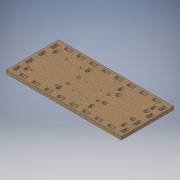
# Autodesk Inventor part: case_base
Saved by Autodesk Inventor 2019 (Build 230136000, 136)
## iProperties
Created: 2019-02-02
Part Number: case_base
Material: MDF Medium Density Fiberboard
Document SubType Name: Modeling
Designer: suchanek
Density: 0.8 g/cm^3
Appearance: Cardboard - Corrugated
Author: suchanek
Autodesk Inventor part; units mm, degrees
ref_plane "YZ Plane" through (0, 0, 0) normal (1, 0, 0) x (0, 1, 0)
ref_plane "XZ Plane" through (0, 0, 0) normal (0, 1, 0) x (-1, 0, 0)
ref_plane "XY Plane" through (0, 0, 0) normal (0, 0, 1) x (1, 0, 0)
sketch "Sketch1" plane through (0, 0, 0) normal (0, 1, 0) x (-1, 0, 0)
  line L0 (110, 50) -> (-110, 50)
  line L1 (-110, 50) -> (-110, -50)
  line L2 (-110, -50) -> (110, -50)
  line L3 (110, -50) -> (110, 50)
  line L4 (110, 50) -> (-110, -50) construction
  line L5 (-110, 50) -> (110, -50) construction
  circle A0 centre (-13.5, 20) radius 0.9
  circle A1 centre (13.5, 20) radius 0.9
  circle A2 centre (13.5, -7) radius 0.9
  circle A3 centre (-13.5, -7) radius 0.9
  line L6 (-13.5, 20) -> (13.5, 20)
  line L7 (13.5, -7) -> (-13.5, -7)
  line L8 (0, 0) -> (4.5236, 0)
  circle A4 centre (28.5, -7) radius 2.6
  circle A5 centre (-28.5, -7) radius 2.6
  circle A6 centre (28.5, 13.5) radius 2.6
  circle A7 centre (-28.5, 13.5) radius 2.6
  line L9 (0, -7) -> (0, -18)
  circle A8 centre (70.5, -25.1) radius 1.6
  circle A9 centre (42.6, -25.1) radius 1.6
  circle A10 centre (85.7, 25.7) radius 1.6
  circle A11 centre (37.5, 27) radius 1.6
  circle A12 centre (-38.5, -16) radius 4
  circle A13 centre (-38.5, 10) radius 4
  circle A14 centre (-92, 10) radius 4
  circle A15 centre (-92, -16) radius 4
  circle A16 centre (31, 28) radius 2.6
  circle A17 centre (31, -28) radius 2.6
  line L10 (0, 0) -> (5.2635, 0)
  circle A18 centre (-31, 28) radius 2.6
  circle A19 centre (-31, -28) radius 2.6
  line L11 (62, 0) -> (62, 7.3763)
  line L12 (-62, 0) -> (-62, 7.3763)
  circle A20 centre (-93, 28) radius 2.6
  circle A21 centre (-93, -28) radius 2.6
  circle A22 centre (93, 28) radius 2.6
  circle A23 centre (93, -28) radius 2.6
  line L13 (106, -42) -> (100, -42)
  line L14 (100, -42) -> (100, -30)
  line L15 (100, -30) -> (106, -30)
  line L16 (106, -30) -> (106, -42)
  line L17 (106, -18) -> (100, -18)
  line L18 (100, -18) -> (100, -6)
  line L19 (100, -6) -> (106, -6)
  line L20 (106, -6) -> (106, -18)
  line L21 (66, -40) -> (54, -40)
  line L22 (54, -40) -> (54, -46)
  line L23 (54, -46) -> (66, -46)
  line L24 (66, -46) -> (66, -40)
  line L25 (42, -40) -> (30, -40)
  line L26 (30, -40) -> (30, -46)
  line L27 (30, -46) -> (42, -46)
  line L28 (42, -46) -> (42, -40)
  line L29 (18, -40) -> (6, -40)
  line L30 (6, -40) -> (6, -46)
  line L31 (6, -46) -> (18, -46)
  line L32 (18, -46) -> (18, -40)
  line L33 (78, -46) -> (90, -46)
  line L34 (90, -46) -> (90, -40)
  line L35 (90, -40) -> (78, -40)
  line L36 (78, -40) -> (78, -46)
  line L37 (-106, -42) -> (-100, -42)
  line L38 (-100, -42) -> (-100, -30)
  line L39 (-100, -30) -> (-106, -30)
  line L40 (-106, -30) -> (-106, -42)
  line L41 (-106, -18) -> (-100, -18)
  line L42 (-100, -18) -> (-100, -6)
  line L43 (-100, -6) -> (-106, -6)
  line L44 (-106, -6) -> (-106, -18)
  line L45 (-66, -40) -> (-54, -40)
  line L46 (-54, -40) -> (-54, -46)
  line L47 (-54, -46) -> (-66, -46)
  line L48 (-66, -46) -> (-66, -40)
  line L49 (-42, -40) -> (-30, -40)
  line L50 (-30, -40) -> (-30, -46)
  line L51 (-30, -46) -> (-42, -46)
  line L52 (-42, -46) -> (-42, -40)
  line L53 (-18, -40) -> (-6, -40)
  line L54 (-6, -40) -> (-6, -46)
  line L55 (-6, -46) -> (-18, -46)
  line L56 (-18, -46) -> (-18, -40)
  line L57 (-78, -46) -> (-90, -46)
  line L58 (-90, -46) -> (-90, -40)
  line L59 (-90, -40) -> (-78, -40)
  line L60 (-78, -40) -> (-78, -46)
  line L61 (106, 42) -> (100, 42)
  line L62 (100, 42) -> (100, 30)
  line L63 (100, 30) -> (106, 30)
  line L64 (106, 30) -> (106, 42)
  line L65 (106, 18) -> (100, 18)
  line L66 (100, 18) -> (100, 6)
  line L67 (100, 6) -> (106, 6)
  line L68 (106, 6) -> (106, 18)
  line L69 (66, 40) -> (54, 40)
  line L70 (54, 40) -> (54, 46)
  line L71 (54, 46) -> (66, 46)
  line L72 (66, 46) -> (66, 40)
  line L73 (42, 40) -> (30, 40)
  line L74 (30, 40) -> (30, 46)
  line L75 (30, 46) -> (42, 46)
  line L76 (42, 46) -> (42, 40)
  line L77 (18, 40) -> (6, 40)
  line L78 (6, 40) -> (6, 46)
  line L79 (6, 46) -> (18, 46)
  line L80 (18, 46) -> (18, 40)
  line L81 (78, 46) -> (90, 46)
  line L82 (90, 46) -> (90, 40)
  line L83 (90, 40) -> (78, 40)
  line L84 (78, 40) -> (78, 46)
  line L85 (-100, 30) -> (-106, 30)
  line L86 (-106, 18) -> (-100, 18)
  line L87 (-100, 18) -> (-100, 6)
  line L88 (-100, 6) -> (-106, 6)
  line L89 (-106, 6) -> (-106, 18)
  line L90 (-106, 42) -> (-100, 42)
  line L91 (-106, 30) -> (-106, 42)
  line L92 (-100, 42) -> (-100, 30)
  line L93 (-90, 40) -> (-78, 40)
  line L94 (-90, 46) -> (-90, 40)
  line L95 (-78, 46) -> (-90, 46)
  line L96 (-78, 40) -> (-78, 46)
  line L97 (-66, 46) -> (-66, 40)
  line L98 (-54, 40) -> (-54, 46)
  line L99 (-54, 46) -> (-66, 46)
  line L100 (-66, 40) -> (-54, 40)
  line L101 (-6, 40) -> (-6, 46)
  line L102 (-18, 40) -> (-6, 40)
  line L103 (-6, 46) -> (-18, 46)
  line L104 (-18, 46) -> (-18, 40)
  line L105 (-30, 40) -> (-30, 46)
  line L106 (-42, 46) -> (-42, 40)
  line L107 (-30, 46) -> (-42, 46)
  line L108 (-42, 40) -> (-30, 40)
  line L109 (93, 25.5) -> (93, 30.5) construction
  line L110 (95.6, 25.5) -> (95.6, 30.5)
  line L111 (90.4, 30.5) -> (90.4, 25.5)
  arc A24 (90.4, 25.5) -> (95.6, 25.5) centre (93, 25.5) ccw
  arc A25 (95.6, 30.5) -> (90.4, 30.5) centre (93, 30.5) ccw
  line L112 (28.4, 25.5) -> (28.4, 30.5)
  line L113 (33.6, 30.5) -> (33.6, 25.5)
  arc A26 (28.4, 25.5) -> (33.6, 25.5) centre (31, 25.5) ccw
  arc A27 (33.6, 30.5) -> (28.4, 30.5) centre (31, 30.5) ccw
  line L114 (-95.6, 25.5) -> (-95.6, 30.5)
  line L115 (-90.4, 30.5) -> (-90.4, 25.5)
  arc A28 (-95.6, 25.5) -> (-90.4, 25.5) centre (-93, 25.5) ccw
  arc A29 (-90.4, 30.5) -> (-95.6, 30.5) centre (-93, 30.5) ccw
  arc A30 (-33.6, 25.5) -> (-28.4, 25.5) centre (-31, 25.5) ccw
  line L116 (-28.4, 25.5) -> (-28.4, 30.5)
  line L117 (-33.6, 30.5) -> (-33.6, 25.5)
  arc A31 (-28.4, 30.5) -> (-33.6, 30.5) centre (-31, 30.5) ccw
  line L118 (93, -25.5) -> (93, -30.5) construction
  line L119 (95.6, -25.5) -> (95.6, -30.5)
  line L120 (90.4, -30.5) -> (90.4, -25.5)
  arc A32 (95.6, -25.5) -> (90.4, -25.5) centre (93, -25.5) ccw
  arc A33 (90.4, -30.5) -> (95.6, -30.5) centre (93, -30.5) ccw
  arc A34 (33.6, -25.5) -> (28.4, -25.5) centre (31, -25.5) ccw
  line L121 (28.4, -25.5) -> (28.4, -30.5)
  line L122 (33.6, -30.5) -> (33.6, -25.5)
  arc A35 (28.4, -30.5) -> (33.6, -30.5) centre (31, -30.5) ccw
  line L123 (-95.6, -25.5) -> (-95.6, -30.5)
  arc A36 (-95.6, -30.5) -> (-90.4, -30.5) centre (-93, -30.5) ccw
  line L124 (-90.4, -30.5) -> (-90.4, -25.5)
  arc A37 (-90.4, -25.5) -> (-95.6, -25.5) centre (-93, -25.5) ccw
  arc A38 (-28.4, -25.5) -> (-33.6, -25.5) centre (-31, -25.5) ccw
  line L125 (-33.6, -30.5) -> (-33.6, -25.5)
  line L126 (-28.4, -25.5) -> (-28.4, -30.5)
  arc A39 (-33.6, -30.5) -> (-28.4, -30.5) centre (-31, -30.5) ccw
  point P0 (0, 0)
  point P1 (0, 0)
  point P2 (31, -28)
  point P3 (-31, -28)
  point P4 (-93, -28)
  point P5 (93, -28)
  dimension "d0" = 100
  dimension "d1" = 220
  dimension "d2" = 27
  dimension "d3" = 1.8
  dimension "d4" = 5.2
  dimension "d5" = 15
  dimension "d6" = 27
  dimension "d7" = 3.2
  dimension "d8" = 5.1
  dimension "d9" = 27.9
  dimension "d10" = 1.3
  dimension "d11" = 50.8
  dimension "d12" = 15.2
  dimension "d13" = 9
  dimension "d14" = 23
  dimension "d16" = 10
  dimension "d19" = 8
  dimension "d22" = 56
  dimension "d23" = 5.2
  dimension "d24" = 62
  dimension "d25" = 186
  dimension "d28" = 10
  dimension "d29" = 16
  dimension "d30" = 92
  dimension "d31" = 6
  dimension "d32" = 4
  dimension "d34" = 6
  dimension "d35" = 12
  dimension "d36" = 12
  dimension "d37" = 12
  dimension "d38" = 6
  dimension "d39" = 12
  dimension "d40" = 12
  dimension "d41" = 12
  dimension "d42" = 12
  dimension "d43" = 12
  dimension "d44" = 12
  dimension "d45" = 12
  dimension "d46" = 6
  dimension "d47" = 4
  dimension "d50" = 2.5
  dimension "d51" = 20
  dimension "d53" = 12
  constraints: 258 end point, 126 symmetric about line, 40 centre point, 32 point on circle, 21 point on line, 15 parallel, 13 equal radius, 11 horizontal, 8 horizontal alignment, 8 midpoint, 7 perpendicular, 6 vertical alignment, 5 tangent, 4 vertical, 3 collinear, 21 other
  measures "d0" distance of L2.end L0.start
  measures "d1" distance of L1.end L2.end
  measures "d2" distance of L7.start L6.end
  measures "d3" diameter of A2
  measures "d4" diameter of A5
  measures "d5" distance of A5.centre L7.end
  measures "d6" distance of L7.start L7.end
  measures "d7" diameter of A9
  measures "d8" horizontal distance of A11.centre A9.centre
  measures "d9" distance of A9.centre A8.centre
  measures "d10" vertical distance of A10.centre A11.centre
  measures "d11" vertical distance of A8.centre A10.centre
  measures "d12" horizontal distance of A10.centre A8.centre
  measures "d13" horizontal distance of A11.centre A6.centre
  measures "d14" distance from line of L0 A11.centre
  measures "d16" horizontal distance of A5.centre A12.centre
  measures "d19" diameter of A12
  measures "d22" distance of A17.centre A16.centre
  measures "d23" diameter of A16
  measures "d24" distance of A16.centre A18.centre
  measures "d25" distance of A20.centre A22.centre
  measures "d28" distance from line of L8 A13.centre
  measures "d29" distance from line of L8 A12.centre
  measures "d30" distance from line of L9 A15.centre
  measures "d31" distance between parallel lines of L18 L20
  measures "d32" distance between parallel lines of L3 L20
  measures "d34" distance between parallel lines of L19 L10
  measures "d35" distance of L19.end L17.start
  measures "d36" distance between parallel lines of L17 L15
  measures "d37" distance of L15.end L13.start
  measures "d38" distance between parallel lines of L30 L9
  measures "d39" distance of L30.end L31.end
  measures "d40" distance between parallel lines of L32 L26
  measures "d41" distance of L25.start L25.end
  measures "d42" distance between parallel lines of L28 L22
  measures "d43" distance of L21.start L21.end
  measures "d44" distance between parallel lines of L24 L36
  measures "d45" distance of L34.end L35.end
  measures "d46" distance of L29.end L30.end
  measures "d47" distance between parallel lines of L2 L31
  measures "d50" distance of A22.centre L109.end
  measures "d51" distance between parallel lines of L8 L6
  measures "d53" vertical distance of A6.centre A26.centre
extrude "Extrusion3" add sketch "Sketch1" along normal blind 6
body "Solid3"
